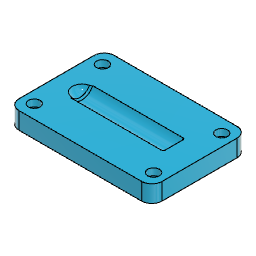
Support_capteur_ILS_KOSMOS3-0 (Autodesk Fusion 360 design; units mm, degrees)
Autodesk Fusion 360 part; units mm, degrees
sketch "Esquisse1" plane through (0, 0, 0) normal (0, 0, 1) x (1, 0, 0)
  line L0 (0, 0) -> (42, 0)
  line L1 (42, 0) -> (42, 28)
  line L2 (42, 28) -> (0, 28)
  line L3 (0, 28) -> (0, 0)
  circle A0 centre (3.5, 24) radius 1.7
  line L4 (21, 28) -> (21, 0) construction
  line L5 (0, 14) -> (42, 14) construction
  circle A1 centre (38.5, 24) radius 1.7
  circle A2 centre (3.5, 4) radius 1.7
  circle A3 centre (38.5, 4) radius 1.7
  circle A4 centre (3.5, 4) radius 3
  circle A5 centre (38.5, 4) radius 3
  circle A6 centre (3.5, 24) radius 3
  circle A7 centre (38.5, 24) radius 3
  point P0 (3.5, 4)
  dimension "d1" = 42
  dimension "d2" = 28
  dimension "d3" = 3.4
  dimension "d4" = 10
  dimension "d5" = 17.5
  dimension "d24" = 6
  constraint horizontal L0
  constraint vertical L1
  constraint horizontal L2
  constraint vertical L3
  constraint coincident L0.start L3.end
  constraint midpoint L2 L4.start
  constraint midpoint L0 L4.end
  constraint midpoint L3 L5.start
  constraint midpoint L1 L5.end
  constraint symmetric A0 L4 A1
  constraint symmetric A0 L5 A2
  constraint symmetric L5 A1 A3
  constraint concentric A2 A4
  constraint symmetric L4 A3.centre P0
  constraint symmetric L4 A4 A5
  constraint symmetric L5 A4 A6
  constraint symmetric L5 A5 A7
  measures "d1" distance of L0.start L0.end
  measures "d2" distance of L0.start L2.end
  measures "d3" diameter of A0
  measures "d4" distance of A0.centre L5
  measures "d5" distance of A0.centre L4
  measures "d24" diameter of A4
extrude "Extrusion1" add sketch "Esquisse1" along normal blind 5 contours L0 L1 L2 L3 | A4 | A5 | A6 | A7
fillet "Congé1" radius 3 4 edges at (0, 0, 2.5) (42, 0, 2.5) (42, 28, 2.5) (0, 28, 2.5)
ref_plane "Plan de construction1" through (21, 0, 0) normal (1, 0, 0) x (0, 1, 0)
sketch "Esquisse2" plane through (21, 0, 0) normal (1, 0, 0) x (0, 1, 0)
  circle A0 centre (14, 6.4) radius 3.45
  dimension "d10" = 6.9
  dimension "d11" = 6.4
  dimension "d12" = 14
  measures "d10" diameter of A0
  measures "d11" vertical distance of origin A0.centre
  measures "d12" horizontal distance of origin A0.centre
extrude "Extrusion2" cut sketch "Esquisse2" along normal blind 13.5 and the other way blind 13.5
ref_plane "Plan de construction2" through (0, 0, 6.4) normal (0, 0, 1) x (1, 0, 0)
sketch "Esquisse3" plane through (0, 0, 6.4) normal (0, 0, 1) x (-1, 0, 0)
  line L0 (-7.5, -10.8468) -> (-7.5, -17.1532)
  line L1 (-7.5, -17.1532) -> (-34.5, -17.1532)
  line L2 (-34.5, -17.1532) -> (-34.5, -10.8468)
  line L3 (-34.5, -10.8468) -> (-7.5, -10.8468)
  arc A0 (-3, -28) -> (0, -25) centre (-3, -25) ccw
  line L4 (0, -25) -> (0, -3)
  arc A1 (0, -3) -> (-3, 0) centre (-3, -3) ccw
  line L5 (-3, 0) -> (-39, 0)
  arc A2 (-39, 0) -> (-42, -3) centre (-39, -3) ccw
  line L6 (-42, -3) -> (-42, -25)
  arc A3 (-42, -25) -> (-39, -28) centre (-39, -25) ccw
  line L7 (-39, -28) -> (-3, -28)
  circle A4 centre (-3.5, -24) radius 1.7
  circle A5 centre (-3.5, -4) radius 1.7
  circle A6 centre (-38.5, -24) radius 1.7
  circle A7 centre (-38.5, -4) radius 1.7
  arc A8 (-7.5, -17.1532) -> (-7.5, -10.8468) centre (-7.5, -14) ccw
  constraint midpoint L0 A8.centre
revolve "Révolution1" cut sketch "Esquisse3" angle 90 about axis through (7.5, 10.8468, 6.4) along (0, -1, 0) contours L0 A8
fillet "Congé2" radius 1 1 edges at (7.5, 14, 3.2468)
fillet "Congé3" radius 0.5 1 edges at (34.5, 14, 2.95)
extrude "Extrusion3" cut sketch "Esquisse1" along normal blind 3 contours A4 | A5 | A6 | A7
equation "d12 = d2 / 2"
equation "d13 = d1 / 2"
